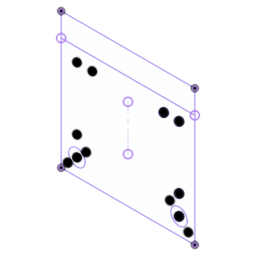
TV Mount (Autodesk Fusion 360 design; units mm, degrees)
Autodesk Fusion 360 part; units mm, degrees
sketch "VESA" plane through (0, 0, 0) normal (0, 1, 0) x (1, 0, 0)
  line L0 (-100, 100) -> (100, 100) construction
  line L1 (100, 100) -> (100, -100) construction
  line L2 (100, -100) -> (-100, -100) construction
  line L3 (-100, -100) -> (-100, 100) construction
  line L4 (-100, 100) -> (100, -100) construction
  line L5 (100, 100) -> (-100, -100) construction
  line L6 (110, -110) -> (-110, -110)
  line L7 (-110, -110) -> (-110, 110)
  line L8 (-110, 110) -> (110, 110)
  line L9 (110, 110) -> (110, -110)
  dimension "d1" = 200
  dimension "d2" = 200
  dimension "d3" = -10
  constraint horizontal L0
  constraint perpendicular L0 L1
  constraint parallel L0 L2
  constraint parallel L1 L3
  constraint coincident L4 origin
  constraint coincident L5 origin
  measures "d1" distance of L1.end L2.end
  measures "d2" distance of L0.end L1.end
sketch "Height Planning" plane through (0, 0, 0) normal (1, 0, 0) x (0, 1, 0)
  line L0 (19, 132.975) -> (37.8, 132.975)
  line L1 (37.8, 132.975) -> (37.8, 44.325)
  line L2 (37.8, 44.325) -> (19, 44.325)
  line L3 (19, 44.325) -> (19, 132.975)
  line L4 (0, 0) -> (37.8, 0)
  line L5 (0, 110) -> (12.1, 110)
  line L6 (12.1, 110) -> (12.1, 74.1)
  line L7 (12.1, 74.1) -> (0, 74.1)
  line L8 (0, 74.1) -> (0, 110)
  line L9 (0, 110) -> (12.1, 110)
  line L10 (12.1, 110) -> (12.1, 112.1)
  line L11 (12.1, 112.1) -> (0, 112.1)
  line L12 (0, 112.1) -> (0, 110)
  line L13 (19, 44.325) -> (37.8, 44.325)
  line L14 (37.8, 44.325) -> (37.8, -44.325)
  line L15 (37.8, -44.325) -> (19, -44.325)
  line L16 (19, -44.325) -> (19, 44.325)
  line L17 (19, -44.325) -> (37.8, -44.325)
  line L18 (37.8, -44.325) -> (37.8, -132.975)
  line L19 (37.8, -132.975) -> (19, -132.975)
  line L20 (19, -132.975) -> (19, -44.325)
  line L21 (19, -84) -> (37.8, -84)
  line L22 (37.8, -84) -> (37.8, -116)
  line L23 (37.8, -116) -> (19, -116)
  line L24 (19, -116) -> (19, -84)
  line L25 (0, -100) -> (19, -100) construction
  line L26 (19, 38.2) -> (17.2, 38.2)
  line L27 (17.2, 38.2) -> (17.2, 74.1)
  line L28 (17.2, 74.1) -> (19, 74.1)
  line L29 (19, 74.1) -> (19, 38.2)
  line L30 (17.2, 74.1) -> (12.1, 74.1) construction
  line L31 (19, -76) -> (16, -76)
  line L32 (16, -76) -> (16, -124)
  line L33 (16, -124) -> (19, -124)
  line L34 (19, -124) -> (19, -76)
  point P0 (0, 110)
  point P1 (0, -110)
  point P2 (0, 100)
  point P3 (19, 0)
  point P4 (0, -100)
  point P5 (19, -100)
  point P6 (16, -100)
  dimension "d4" = 12.1
  dimension "d6" = 12.1
  dimension "d7" = 38
  dimension "d8" = 18.8
  dimension "d9" = 88.65
  dimension "d11" = 32
  dimension "d12" = 1.8
  dimension "d13" = 5.1
  dimension "d27" = 3
  dimension "d28" = 48
  constraint horizontal L0
  constraint vertical L1
  constraint horizontal L2
  constraint vertical L3
  constraint coincident L4.start origin
  constraint perpendicular L1 L4
  constraint horizontal L5
  constraint vertical L6
  constraint horizontal L7
  constraint vertical L8
  constraint coincident P0 L5.start
  constraint horizontal L9
  constraint vertical L10
  constraint horizontal L11
  constraint vertical L12
  constraint coincident L5.end L10
  constraint horizontal L13
  constraint vertical L14
  constraint horizontal L15
  constraint vertical L16
  constraint coincident L1.end L14
  constraint equal L1 L14
  constraint midpoint L16 P3
  constraint coincident L4 P3
  constraint coincident L4.end L14
  constraint horizontal L17
  constraint vertical L18
  constraint horizontal L19
  constraint vertical L20
  constraint equal L14 L18
  constraint coincident L14.end L15.start
  constraint horizontal L21
  constraint vertical L22
  constraint horizontal L23
  constraint vertical L24
  constraint coincident L18 L22.end
  constraint coincident L20 L21.start
  constraint midpoint L24 P5
  constraint coincident P4 L25.start
  constraint coincident P5 L25.end
  constraint horizontal L25
  constraint horizontal L26
  constraint vertical L27
  constraint horizontal L28
  constraint vertical L29
  constraint coincident L16 L26.start
  constraint horizontal L30
  constraint equal L6 L27
  constraint horizontal L31
  constraint vertical L32
  constraint horizontal L33
  constraint vertical L34
  constraint coincident L20 L31.start
  constraint midpoint L32 P6
  constraint coincident L25 P6
  measures "d4" distance of P0 L5.end
  measures "d6" distance of L11.end P2
  measures "d7" distance of L6.end L10.end
  measures "d8" distance of L0.start L0.end
  measures "d9" distance of L0.end L1.end
  measures "d11" distance of L21.end L22.end
  measures "d12" distance of L27.end L28.end
  measures "d13" distance of L6.end L27.end
  measures "d27" distance of L31.start L31.end
  measures "d28" distance of L31.end L32.end
sketch "Back Board Planning" plane through (0, 0, 0) normal (0, 1, 0) x (1, 0, 0)
  line L0 (-100, 84) -> (100, 84) construction
  line L1 (100, 84) -> (100, 116) construction
  line L2 (100, 116) -> (-100, 116) construction
  line L3 (-100, 116) -> (-100, 84) construction
  circle A0 centre (-100, 100) radius 16
  circle A1 centre (100, 100) radius 16
  line L4 (-131, 132.975) -> (131, 132.975)
  line L5 (131, 132.975) -> (131, -132.975)
  line L6 (131, -132.975) -> (-131, -132.975)
  line L7 (-131, -132.975) -> (-131, 132.975)
  line L8 (-131, 44.325) -> (131, 44.325)
  line L9 (-131, -44.325) -> (131, -44.325)
  line L10 (-100, -100) -> (-100, -112.1) construction
  line L11 (-100, -100) -> (-110, -100) construction
  line L12 (-110, -112.1) -> (-60, -112.1) construction
  line L13 (-60, -112.1) -> (-60, -87.1) construction
  line L14 (-60, -87.1) -> (-110, -87.1) construction
  line L15 (-110, -87.1) -> (-110, -112.1) construction
  line L16 (-60, -87.1) -> (-110, -87.1) construction
  line L17 (-110, -87.1) -> (-110, -74.1) construction
  line L18 (-110, -74.1) -> (-60, -74.1) construction
  line L19 (-60, -74.1) -> (-60, -87.1) construction
  line L20 (-110, -74.1) -> (-60, -74.1) construction
  line L21 (-60, -74.1) -> (-60, -49.1) construction
  line L22 (-60, -49.1) -> (-110, -49.1) construction
  line L23 (-110, -49.1) -> (-110, -74.1) construction
  line L24 (-110, -61.2) -> (-60, -61.2) construction
  line L25 (-100, -100) -> (-100, 100) construction
  line L26 (-100, -100) -> (-70, -100) construction
  line L27 (-70, -100) -> (-70, -61.2) construction
  line L28 (-70, -61.2) -> (-100, -61.2) construction
  line L29 (-100, -61.2) -> (-100, -100) construction
  line L30 (0, 0) -> (-131, 0) construction
  line L31 (0, 44.325) -> (0, -44.325) construction
  line L32 (-131, -87.025) -> (131, -87.025)
  point P0 (-100, -100)
  point P1 (-100, 100)
  point P2 (100, 100)
  point P3 (100, -100)
  point P4 (0, 84)
  point P5 (0, 116)
  point P6 (0, 84)
  point P7 (0, -132.975)
  point P8 (0, -132.975)
  point P9 (0, 132.975)
  point P10 (0, 44.325)
  point P11 (0, -44.325)
  point P12 (0, -44.325)
  point P13 (-100, -61.2)
  point P14 (-70, -100)
  point P15 (-70, -61.2)
  point P16 (-100, 61.2)
  point P17 (100, -61.2)
  point P18 (70, -61.2)
  point P19 (100, 61.2)
  dimension "d14" = 262
  dimension "d15" = 12.1
  dimension "d16" = 10
  dimension "d17" = 50
  dimension "d18" = 25
  dimension "d19" = 13
  dimension "d20" = 25
  dimension "d21" = 12.1
  dimension "d22" = 30
  dimension "d53" = 220
  constraint horizontal L0
  constraint vertical L1
  constraint horizontal L2
  constraint vertical L3
  constraint coincident P2 L1
  constraint coincident P1 L3
  constraint coincident L0 P6
  constraint coincident P5 L2
  constraint coincident P1 A0.centre
  constraint coincident L0.start A0
  constraint coincident P2 A1.centre
  constraint coincident L0.end A1
  constraint horizontal L4
  constraint vertical L5
  constraint horizontal L6
  constraint vertical L7
  constraint midpoint L6 P8
  constraint coincident L4 P9
  constraint coincident P8 P7
  constraint coincident L7 L8.start
  constraint coincident L5 L8.end
  constraint perpendicular L5 L8
  constraint coincident P10 L8
  constraint coincident L7 L9.start
  constraint coincident L5 L9.end
  constraint perpendicular L5 L9
  constraint coincident L9 P12
  constraint coincident P0 L10.start
  constraint vertical L10
  constraint perpendicular L10 L11
  constraint horizontal L12
  constraint vertical L13
  constraint horizontal L14
  constraint vertical L15
  constraint coincident L10.end L12
  constraint coincident L11.end L15
  constraint horizontal L16
  constraint vertical L17
  constraint horizontal L18
  constraint vertical L19
  constraint coincident L14.end L17
  constraint horizontal L20
  constraint vertical L21
  constraint horizontal L22
  constraint vertical L23
  constraint coincident L18.end L21
  constraint coincident L23 L24.start
  constraint coincident L21 L24.end
  constraint perpendicular L21 L24
  constraint coincident L24 P13
  constraint coincident P13 L25
  constraint horizontal L26
  constraint vertical L27
  constraint horizontal L28
  constraint vertical L29
  constraint coincident P13 L28.end
  constraint coincident P14 L26.end
  constraint coincident P15 L27.end
  constraint coincident L30.start origin
  constraint midpoint L7 L30.end
  constraint symmetric P13 L30 P16
  constraint coincident P10 L31.start
  constraint coincident P12 P11
  constraint symmetric P13 L31 P17
  constraint symmetric P15 L31 P18
  constraint symmetric P16 L31 P19
  constraint coincident L7 L32.start
  constraint coincident L5 L32.end
  constraint perpendicular L5 L32
  measures "d14" distance of L4.start L4.end
  measures "d15" distance of P0 L10.end
  measures "d16" distance of P0 L11.end
  measures "d17" distance of L12.start L12.end
  measures "d18" distance of L12.start L14.end
  measures "d19" distance of L13.end L18.end
  measures "d20" distance of L17.end L22.end
  measures "d21" distance of L22 L24
  measures "d22" distance of P0 P14
  measures "d53" distance of L4.end L32.end
sketch "Bracket Planning" plane through (0, 0, 0) normal (0, 1, 0) x (1, 0, 0)
  circle A0 centre (-100, 100) radius 16 construction
  circle A1 centre (100, 100) radius 16 construction
  line L0 (-82, 82) -> (-118, 82) construction
  line L1 (-118, 82) -> (-118, 118) construction
  line L2 (-118, 118) -> (-82, 118) construction
  line L3 (-82, 118) -> (-82, 82) construction
  line L4 (-82, 82) -> (-118, 118) construction
  line L5 (-118, 82) -> (-82, 118) construction
  line L6 (0, 44.325) -> (0, -44.325) construction
  circle A2 centre (-100, 100) radius 14.5
  line L7 (-124, 124) -> (-76, 124) construction
  line L8 (-76, 124) -> (-76, 76) construction
  line L9 (-76, 76) -> (-124, 76) construction
  line L10 (-124, 76) -> (-124, 124) construction
  arc A3 (-82, 76) -> (-76, 82) centre (-82, 82) ccw
  arc A4 (-118, 124) -> (-124, 118) centre (-118, 118) ccw
  arc A5 (-124, 100) -> (-100, 76) centre (-100, 100) ccw
  line L11 (-124, 100) -> (-124, 118)
  line L12 (-82, 76) -> (-100, 76)
  arc A6 (-76, 100) -> (-100, 124) centre (-100, 100) ccw
  line L13 (-76, 82) -> (-76, 100)
  line L14 (-100, 124) -> (-118, 124)
  point P0 (-100, 100)
  point P1 (100, 100)
  point P2 (-100, 100)
  point P3 (-82, 82)
  point P4 (-118, 118)
  dimension "d24" = 36
  dimension "d25" = 29
  dimension "d26" = -6
  constraint horizontal L0
  constraint perpendicular L0 L1
  constraint parallel L0 L2
  constraint parallel L1 L3
  constraint coincident L4 P2
  constraint coincident L5 P2
  constraint coincident P2 P0
  constraint coincident P3 L0.start
  constraint coincident P4 L1.end
  constraint coincident L8 A3.end
  constraint coincident L9 A3.start
  constraint horizontal P3 A3.end
  constraint symmetric L5 A3.start A4.end
  constraint symmetric L5 A3.end A4.start
  constraint symmetric L5 A3 A4
  constraint midpoint L9 A5.end
  constraint midpoint L10 A5.start
  constraint symmetric L4 A3.start A3.end
  constraint symmetric L4 A4.end A4.start
  constraint symmetric L4 A5.start A6.end
  constraint symmetric L4 A5.end A6.start
  constraint symmetric L4 A5 A6
  measures "d24" distance of L0.end P4
  measures "d25" diameter of A2
extrude "Extrude1" add sketch "Bracket Planning" along normal up to surface (3 mm away) from surface at 16 makes body 1
extrude "Extrude2" add sketch "Height Planning" along normal mid plane 220 separate body contours L5 L9 L10 L11 L12 | L5 L6 L7 L8 L9 makes body 2
sketch "Bracket Holes" plane through (0, 16, 0) normal (0, -1, 0) x (1, 0, 0)
  circle A0 centre (-100, -100) radius 14.5
  arc A1 (-76, -82) -> (-82, -76) centre (-82, -82) ccw
  line L0 (-82, -76) -> (-100, -76)
  arc A2 (-100, -76) -> (-124, -100) centre (-100, -100) ccw
  line L1 (-124, -100) -> (-124, -118)
  arc A3 (-124, -118) -> (-118, -124) centre (-118, -118) ccw
  line L2 (-118, -124) -> (-100, -124)
  arc A4 (-100, -124) -> (-76, -100) centre (-100, -100) ccw
  line L3 (-76, -100) -> (-76, -82)
  point P0 (-82, -82)
  point P1 (-118, -118)
hole "Hole1" at (-82, 16, -82) at (-118, 16, -118) direction (0, 1, 0) diameter 3.7 depth 35 tip angle 118 countersink diameter 7.2 countersink angle 82 bodies 1
extrude "Extrude3" add sketch "Height Planning" along normal mid plane 262 separate body contours L0 L1 L2 L3 L13 L29 | L2 L4 L13 L14 L16 L29 | L4 L14 L15 L16 L17 | L15 L17 L18 L20 L21 L34 | L18 L20 L21 L22 L23 L24 L34 | L18 L19 L20 L23 L34 makes body 3
mirror "Mirror1" about plane through (0, 0, 0) normal (1, 0, 0) of bodies 1 makes body 4
extrude "Extrude4" cut sketch "Back Board Planning" along normal up to surface (37.8 mm away) contours A0 | A1 bodies 3
extrude "Extrude6" cut sketch "Back Board Planning" along normal through all contours L5 L6 L7 L32 bodies 3
sketch "Sketch7" plane through (0, 0, 0) normal (1, 0, 0) x (0, 1, 0)
  line L0 (37.8, 87.025) -> (19, 87.025)
  line L1 (19, 87.025) -> (19, -132.975)
  line L2 (19, -132.975) -> (37.8, -132.975)
  line L3 (37.8, -132.975) -> (37.8, 87.025)
  line L4 (19.1, -132.875) -> (37.7, -132.875)
  line L5 (37.7, -132.875) -> (37.7, 86.925)
  line L6 (37.7, 86.925) -> (19.1, 86.925)
  line L7 (19.1, 86.925) -> (19.1, -132.875)
  line L8 (0, 49.1) -> (19, 49.1) construction
  line L9 (17.1, 49.1) -> (17.1, 92.025)
  line L10 (17.1, 92.025) -> (36.7, 92.025)
  line L11 (36.7, 92.025) -> (36.7, 87.025)
  line L12 (17.1, 49.1) -> (19, 49.1)
  point P0 (0, 49.1)
  point P1 (17.2, 74.1)
  dimension "d54" = -0.1
  dimension "d55" = 1
  dimension "d56" = 5
  dimension "d57" = 0.1
  constraint coincident P0 L8.start
  constraint coincident L1 L8.end
  constraint perpendicular L7 L8
  constraint coincident L8 L9.start
  constraint perpendicular L8 L9
  constraint perpendicular L9 L10
  constraint coincident L0 L11.end
  constraint perpendicular L0 L11
  measures "d55" distance of L5 L11.end
  measures "d56" distance of L10.end L11.end
  measures "d57" distance of L9 P1
extrude "Extrude7" add sketch "Sketch7" along normal mid plane 262 separate body contours L0 L1 L9 L10 L11 L12 makes body 5
sketch "holes 4 back plate" plane through (0, 0, 0) normal (0, 1, 0) x (1, 0, 0)
  line L0 (131, -132.975) -> (-131, -132.975)
  line L1 (-131, -132.975) -> (-131, 132.975)
  line L2 (131, 132.975) -> (131, -132.975)
  line L3 (-131, 132.975) -> (131, 132.975)
  line L4 (0, 44.325) -> (0, -44.325)
  line L5 (-131, -87.025) -> (131, -87.025)
  circle A0 centre (-100, 100) radius 16
  circle A1 centre (100, 100) radius 16
  line L6 (-118, 120.5) -> (-118, 115.5)
  line L7 (-120.5, 118) -> (-115.5, 118)
  line L8 (-84.5, 82) -> (-79.5, 82)
  line L9 (-82, 84.5) -> (-82, 79.5)
  line L10 (-100, 63.7) -> (-100, 58.7)
  line L11 (-102.5, 61.2) -> (-97.5, 61.2)
  line L12 (-100, -58.7) -> (-100, -63.7)
  line L13 (-97.5, -61.2) -> (-102.5, -61.2)
  line L14 (-70, -58.7) -> (-70, -63.7)
  line L15 (-72.5, -61.2) -> (-67.5, -61.2)
  line L16 (120.5, 118) -> (115.5, 118)
  line L17 (82, 84.5) -> (82, 79.5)
  line L18 (84.5, 82) -> (79.5, 82)
  line L19 (100, 63.7) -> (100, 58.7)
  line L20 (102.5, 61.2) -> (97.5, 61.2)
  line L21 (100, -58.7) -> (100, -63.7)
  line L22 (97.5, -61.2) -> (102.5, -61.2)
  line L23 (72.5, -61.2) -> (67.5, -61.2)
  line L24 (70, -58.7) -> (70, -63.7)
  line L25 (118, 120.5) -> (118, 115.5)
  line L26 (-100, 102.5) -> (-100, 97.5)
  line L27 (-102.5, 100) -> (-97.5, 100)
  line L28 (102.5, 100) -> (97.5, 100)
  line L29 (100, 102.5) -> (100, 97.5)
  point P0 (100, 61.2)
  point P1 (-100, 61.2)
  point P2 (-82, 82)
  point P3 (-118, 118)
  point P4 (-100, 100)
  point P5 (-100, -61.2)
  point P6 (-70, -61.2)
  point P7 (70, -61.2)
  point P8 (100, -61.2)
  point P9 (82, 82)
  point P10 (100, 100)
  point P11 (118, 118)
  dimension "d67" = 5
  constraint symmetric P2 L4 P9
  constraint symmetric P3 L4 P11
  constraint symmetric P4 L4 P10
  constraint parallel L1 L6
  constraint midpoint P3 L6
  constraint horizontal L7
  constraint equal L6 L7
  constraint midpoint P3 L7
  constraint horizontal L8
  constraint perpendicular L8 L9
  constraint equal L7 L9
  constraint equal L8 L9
  constraint midpoint P2 L8
  constraint midpoint P2 L9
  constraint vertical L10
  constraint horizontal L11
  constraint equal L8 L11
  constraint equal L10 L11
  constraint midpoint P1 L11
  constraint midpoint P1 L10
  constraint vertical L12
  constraint horizontal L13
  constraint equal L11 L12
  constraint equal L12 L13
  constraint midpoint P5 L13
  constraint midpoint P5 L12
  constraint vertical L14
  constraint equal L12 L14
  constraint perpendicular L14 L15
  constraint equal L14 L15
  constraint midpoint P6 L14
  constraint midpoint P6 L15
  constraint symmetric L4 L7.start L16.start
  constraint symmetric L4 L7.end L16.end
  constraint symmetric L4 L8.start L18.start
  constraint symmetric L4 L8.end L18.end
  constraint symmetric L4 L9.start L17.start
  constraint symmetric L4 L9.end L17.end
  constraint symmetric L4 L10.start L19.start
  constraint symmetric L4 L10.end L19.end
  constraint symmetric L4 L11.start L20.start
  constraint symmetric L4 L11.end L20.end
  constraint symmetric L4 L12.start L21.start
  constraint symmetric L4 L12.end L21.end
  constraint symmetric L4 L13.start L22.start
  constraint symmetric L4 L13.end L22.end
  constraint symmetric L4 L14.start L24.start
  constraint symmetric L4 L14.end L24.end
  constraint symmetric L4 L15.start L23.start
  constraint symmetric L4 L15.end L23.end
  constraint symmetric L4 L6.start L25.start
  constraint symmetric L4 L6.end L25.end
  constraint vertical L26
  constraint perpendicular L26 L27
  constraint equal L6 L26
  constraint equal L26 L27
  constraint midpoint P4 L27
  constraint midpoint P4 L26
  constraint symmetric L4 L26.start L29.start
  constraint symmetric L4 L26.end L29.end
  constraint symmetric L4 L27.start L28.start
  constraint symmetric L4 L27.end L28.end
  measures "d67" distance of L6.start L6.end
hole "Hole3" at (-100, 0, 61.2) at (100, 0, 61.2) at (-100, 0, -61.2) at (100, 0, -61.2) direction (0, 1, 0) diameter 4.5 end through all bodies 3 5
hole "Hole4" at (-70, 0, 61.2) at (70, 0, 61.2) direction (0, 1, 0) diameter 3.7 end through all bodies 5
hole "Hole5" at (-70, 0, 61.2) at (-82, 0, -82) at (-118, 0, -118) at (70, 0, 61.2) at (82, 0, -82) at (118, 0, -118) direction (0, 1, 0) diameter 2.5 end through all bodies 5 3
sketch "holes 4 front plate" plane through (0, 0, 0) normal (0, -1, 0) x (1, 0, 0)
  line L0 (-110, 74.1) -> (110, 74.1)
  line L1 (110, 74.1) -> (110, 112.1)
  line L2 (110, 112.1) -> (-110, 112.1)
  line L3 (-110, 112.1) -> (-110, 74.1)
  line L4 (0, -44.325) -> (0, 44.325)
  line L5 (-100, 97.5) -> (-100, 102.5)
  line L6 (-97.5, 100) -> (-102.5, 100)
  line L7 (-72.5, 100) -> (-67.5, 100)
  line L8 (-70, 97.5) -> (-70, 102.5)
  line L9 (72.5, 100) -> (67.5, 100)
  line L10 (70, 97.5) -> (70, 102.5)
  line L11 (97.5, 100) -> (102.5, 100)
  line L12 (100, 97.5) -> (100, 102.5)
  point P0 (-100, 100)
  point P1 (-70, 100)
  point P2 (100, 100)
  point P3 (70, 100)
  dimension "d66" = 5
  constraint symmetric P0 L4 P2
  constraint symmetric P1 L4 P3
  constraint vertical L5
  constraint midpoint P0 L5
  constraint perpendicular L5 L6
  constraint midpoint P0 L6
  constraint equal L5 L6
  constraint horizontal L7
  constraint midpoint P1 L7
  constraint equal L6 L7
  constraint perpendicular L7 L8
  constraint midpoint P1 L8
  constraint equal L7 L8
  constraint symmetric L4 L5.start L12.start
  constraint symmetric L4 L5.end L12.end
  constraint symmetric L4 L6.start L11.start
  constraint symmetric L4 L6.end L11.end
  constraint symmetric L4 L7.start L9.start
  constraint symmetric L4 L7.end L9.end
  constraint symmetric L4 L8.start L10.start
  constraint symmetric L4 L8.end L10.end
  measures "d66" distance of L5.start L5.end
hidden bodies 1 2 3 4 5
equation "d28 = 36 mm + 12 mm"
equation "d62 = 3.4 mm + 0.3 mm"
named bodies: "Bracket", "Front Plate", "Back Plate", "Bracket (1)", "Back Spacer"
